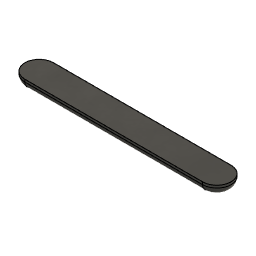
SKUF-ASSEMBLY (Autodesk Fusion 360 design; units mm, degrees)
part number: RW_PARAMETRIC_BUMPON
Autodesk Fusion 360 part; units mm, degrees
sketch "SKUF" plane through (0, 0, 0) normal (0, 1, 0) x (1, 0, 0)
  line L0 (-18, 2.9) -> (18, 2.9)
  line L1 (18, 2.9) -> (18, -2.9) construction
  line L2 (18, -2.9) -> (-18, -2.9)
  line L3 (-18, -2.9) -> (-18, 2.9) construction
  arc A0 (-18, 2.9) -> (-18, -2.9) centre (-18, 0) ccw
  arc A1 (18, -2.9) -> (18, 2.9) centre (18, 0) ccw
  line L4 (0, 2.9) -> (0, -2.9) construction
  line L5 (-20.9, 0) -> (20.9, 0) construction
  dimension "d1" = 5.8
  dimension "d2" = 36
  dimension "d10" = 41.6
  constraint horizontal L0
  constraint vertical L1
  constraint horizontal L2
  constraint vertical L3
  constraint midpoint L3 A0.centre
  constraint midpoint L1 A1.centre
  constraint midpoint L4 origin
  constraint vertical L4
  constraint midpoint L0 L4.start
  constraint midpoint L2 L4.end
  constraint horizontal L5
  constraint coincident A0 L5.start
  constraint coincident A1 L5.end
  constraint coincident origin L5
  measures "d1" distance of L0.start L2.end
  measures "d2" distance of L0.start L0.end
extrude "Basic shape extrusion" add sketch "SKUF" against normal blind 2
fillet "Bottom fillet" radius 1.5 4 edges at (0, -2, -2.9) (20.9, -2, 0) (0, -2, 2.9) (-20.9, -2, 0)
equation "d1 = SKUF_Z"
equation "d2 = SKUF_X"
equation "d3 = -SKUF_Y"
equation "d5 = SKUF_STICK_OUT"
equation "SKUF_X = 36 mm" comment "42mm X slot"
equation "SKUF_Y = 2.00 mm"
equation "SKUF_Z = 5.80 mm" comment "6mm Z slot"
equation "SKUF_SLOT_Y = 0.50 mm" comment "0.5mm Y slot"
equation "SKUF_STICK_OUT = SKUF_Y - SKUF_SLOT_Y"
named bodies: "SKUF"
